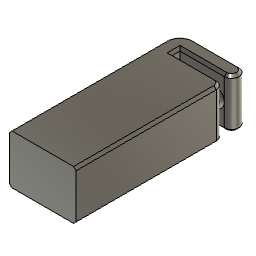
ErgoDonk Solering jig v19 (Autodesk Fusion 360 design; units mm, degrees)
Autodesk Fusion 360 part; units mm, degrees
sketch "Sketch2" plane through (0, 0, 0) normal (0, 0, 1) x (1, 0, 0)
  line L0 (-0.6794, 183.904) -> (9.8206, 183.904)
  line L1 (9.8206, 183.904) -> (9.8206, 182.304)
  line L2 (9.8206, 182.304) -> (-0.6794, 182.304)
  line L3 (-0.6794, 182.304) -> (-0.6794, 183.904)
  line L4 (12.8206, 179.304) -> (-3.6794, 179.304)
  line L5 (-3.6794, 179.304) -> (-3.6794, 186.904)
  line L6 (-3.6794, 186.904) -> (12.8206, 186.904)
  line L7 (12.8206, 186.904) -> (12.8206, 179.304)
  line L8 (-3.6794, 182.304) -> (12.8206, 182.304)
  line L9 (12.8206, 182.304) -> (12.8206, 152.304)
  line L10 (12.8206, 152.304) -> (-3.6794, 152.304)
  line L11 (-3.6794, 152.304) -> (-3.6794, 182.304)
  line L12 (9.8206, 186.904) -> (9.8206, 152.304)
  dimension "d63" = 10.5
  dimension "d64" = 1.6
  dimension "d66" = 30
  constraint horizontal L0
  constraint vertical L1
  constraint horizontal L2
  constraint vertical L3
  constraint horizontal L8
  constraint vertical L9
  constraint horizontal L10
  constraint vertical L11
  constraint coincident L5 L8.start
  constraint coincident L6 L12.start
  constraint coincident L10 L12.end
  constraint perpendicular L10 L12
  constraint collinear L7 L9
  constraint collinear L1 L12
  measures "d63" distance of L0.start L0.end
  measures "d64" distance of L0.start L2.end
  measures "d66" distance of L8.start L10.end
extrude "Extrude12" add sketch "Sketch2" along normal blind 10 contours L0 L3 L5 L6 L8 L12 | L2 L4 L5 L8 L11 L12 | L4 L10 L11 L12
fillet "Fillet1" radius 1.5 3 edges at (9.8206, 183.904, 5) (9.8206, 186.904, 5) (9.8206, 182.304, 5)
fillet "Fillet2" radius 3 1 edges at (-3.6794, 186.904, 5)
chamfer "Chamfer2" distance 0.5 angle 45 18 edges at (-3.6794, 168.104, 0) (-2.8008, 186.0253, 0) (3.8206, 186.904, 0) (9.8206, 185.404, 0) (3.8206, 183.904, 0) (-0.6794, 183.104, 0) (3.8206, 182.304, 0) (9.3812, 181.8646, 0) (9.8206, 166.554, 0) (-3.6794, 168.104, 10) (-2.8008, 186.0253, 10) (3.8206, 186.904, 10) (9.8206, 185.404, 10) (3.8206, 183.904, 10) (3.8206, 182.304, 10) (9.3812, 181.8646, 10) (9.8206, 166.554, 10) (-0.6794, 183.104, 10)
sketch "Sketch3" plane through (0, 183.904, 0) normal (0, -1, 0) x (1, 0, 0)
  line L0 (8.3206, 9.5) -> (-0.6794, 9.5)
  line L1 (-0.6794, 9.5) -> (-0.6794, 0.5)
  line L2 (-0.6794, 0.5) -> (8.3206, 0.5)
  line L3 (8.3206, 0.5) -> (8.3206, 9.5)
  line L4 (-0.6794, 9.5) -> (8.3206, 0.5) construction
  line L5 (-0.6794, 0.5) -> (8.3206, 9.5) construction
  line L6 (8.3206, 5) -> (3.8206, 5) construction
  circle A0 centre (6.3206, 5) radius 2
  dimension "d75" = 4
  constraint coincident L0.end L1.start
  constraint coincident L2.end L3.start
  constraint coincident L1.end L2.start
  constraint coincident L0.start L3.end
  constraint midpoint L3 L6.start
  constraint midpoint L5 L6.end
  constraint coincident L6.start A0
  measures "d75" diameter of A0
extrude "Extrude13" add sketch "Sketch3" along normal blind 0.5 contours A0
chamfer "Chamfer3" distance 0.5 angle 45 1 edges at (4.4559, 183.404, 4.2768)
equation "d63 = slot_depth"
equation "d64 = pcb_thickness"
equation "d65 = -wall_thickness"
equation "d66 = leg_height"
equation "d67 = leg_thickness"
equation "leg_height = 30 mm"
equation "pcb_thickness = 1.6 mm"
equation "wall_thickness = 3 mm"
equation "slot_depth = 10.5 mm"
equation "leg_thickness = 10 mm"
named bodies: "ergodonk_zero_workholding_feet"
